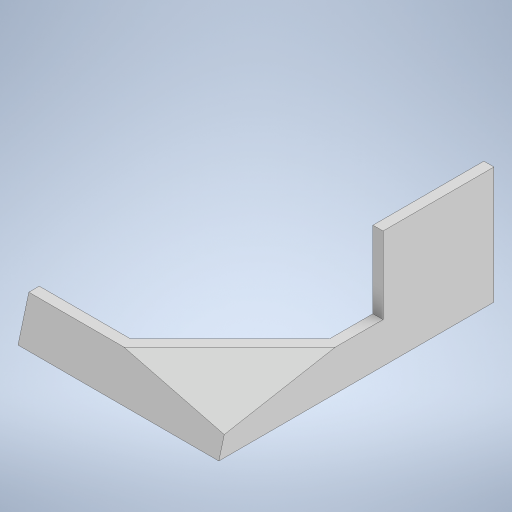
# Autodesk Inventor part: body
Saved by Autodesk Inventor 2024 (Build 280153000, 153)
## iProperties
Created: 2024-01-31
Part Number: body
Material: Všeobecné
Document SubType Name: Modeling
Designer: Simak
Density: 1 g/cm^3
Appearance: Výchozí
Author: Simak
Autodesk Inventor part; units mm, degrees
ref_plane "YZ Plane" through (0, 0, 0) normal (1, 0, 0) x (0, 1, 0)
ref_plane "XZ Plane" through (0, 0, 0) normal (0, 1, 0) x (-1, 0, 0)
ref_plane "XY Plane" through (0, 0, 0) normal (0, 0, 1) x (1, 0, 0)
sketch "Náčrt2" plane through (0, 0, 0) normal (0, 1, 0) x (-1, 0, 0)
  line L0 (0, 49.75) -> (-49.75, 49.75)
  line L1 (-49.75, 49.75) -> (-49.75, -49.75)
  line L2 (-49.75, -49.75) -> (0, -49.75)
  line L3 (-49.75, 49.75) -> (0, 0) construction
  line L4 (0, 0) -> (-49.75, -49.75) construction
  line L5 (-47.25, 49.75) -> (-47.25, -19.75)
  line L6 (-47.25, -19.75) -> (-49.75, -19.75)
  line L7 (0, 49.75) -> (0, -49.75)
  dimension "d0" = 99.5
  dimension "d1" = 69.5
  dimension "d2" = 2.5
  constraints: 16 end point, 5 perpendicular, 2 point on line, 2 vertical, 2 vertical alignment, 1 horizontal
  measures "d0" distance of L0.end L1.end
  measures "d1" distance of L5.start L5.end
  measures "d2" distance of L5.end L6.end
extrude "Vysunutí1" add sketch "Náčrt2" along normal blind 10 contours L5 L6 L1 L0
sketch "Náčrt3" plane through (49.75, 0, 49.75) normal (1, 0, 0) x (0, 0, -1)
  line L0 (69.5, 0) -> (0, 0) projected
  line L1 (69.5, 10) -> (0, 10) projected
  line L2 (0, 0) -> (0, 10) projected
  line L3 (0, 0) -> (0, -5)
  line L4 (0, -5) -> (69.5, -5) construction
  line L5 (69.5, -5) -> (69.5, 0) construction
  line L6 (0, -5) -> (4.0192, 10)
  point P0 (49.75, 0)
  point P1 (1.3397, 0)
  dimension "d8" = 5
  dimension "d9" = 75
  constraints: 8 end point, 2 perpendicular, 1 point on line, 1 vertical
  measures "d8" distance of L4.end L0.start
  measures "d9" angle of L4 L6
extrude "Vysunutí2" cut sketch "Náčrt3" against normal blind 10 contours L0 L2 L1 L6
sketch "Náčrt4" plane through (49.75, 0, -19.75) normal (1, 0, 0) x (0, 0, -1)
  line L0 (0, 10) -> (-65.4808, 10) projected
  line L1 (-62.8926, 10) -> (-65.5721, 0)
  line L2 (0, 0) -> (-68.1603, 0) projected
  line L3 (-65.4808, 10) -> (-68.1603, 0) projected
  point P0 (-19.75, 0)
  dimension "d10" = 2.5
  constraints: 2 end point, 2 point on line, 1 parallel
  measures "d10" distance between parallel lines of L3 L1
extrude "Vysunutí3" add sketch "Náčrt4" against normal up to surface (49.75 mm away)
sketch "Náčrt5" plane through (49.75, 0, -19.75) normal (1, 0, 0) x (0, 0, -1)
  line L0 (-65.4808, 10) -> (0, 10) projected
  line L1 (-27.4808, 10) -> (0, 10)
  line L2 (0, 10) -> (0, 29)
  line L3 (0, 29) -> (-27.4808, 29)
  line L4 (-27.4808, 29) -> (-27.4808, 10)
  point P0 (-19.75, 0)
  dimension "d13" = 38
  dimension "d14" = 19
  constraints: 8 end point, 2 parallel, 1 horizontal, 1 perpendicular, 1 point on line
  measures "d13" distance from line of L4 L0.start
  measures "d14" distance of L3.end L1.start
extrude "Vysunutí4" add sketch "Náčrt5" against normal up to surface (2.5 mm away)
sketch "Náčrt6" plane through (47.25, 0, -19.75) normal (-1, 0, 0) x (0, 0, 1)
  line L0 (65.5721, 0) -> (62.8926, 10) projected
  line L1 (57.5721, 1) -> (65.5721, 1)
  line L2 (65.5721, 1) -> (65.5721, 0)
  line L3 (65.5721, 0) -> (57.5721, 0)
  line L4 (57.5721, 0) -> (57.5721, 1)
  point P0 (19.75, 0)
  dimension "d17" = 1
  dimension "d18" = 8
  constraints: 8 end point, 2 parallel, 1 horizontal, 1 perpendicular
  measures "d17" distance of L3.end L1.start
  measures "d18" distance of L1.start L1.end
extrude "Vysunutí5" add sketch "Náčrt6" along normal up to surface (47.25 mm away)
sketch "Náčrt7" plane through (47.25, 0, -19.75) normal (-1, 0, 0) x (0, 0, 1)
  line L0 (62.8926, 10) -> (65.3041, 1) projected
  line L1 (64.7682, 3) -> (65.3041, 3)
  line L2 (65.3041, 3) -> (65.3041, 1)
  line L3 (65.3041, 1) -> (64.7682, 1)
  line L4 (64.7682, 1) -> (64.7682, 3)
  point P0 (19.75, 0)
  dimension "d21" = 2
  constraints: 8 end point, 2 parallel, 1 horizontal, 1 perpendicular, 1 point on line
  measures "d21" distance of L3.end L1.start
extrude "Vysunutí6" cut sketch "Náčrt7" along normal up to surface (47.25 mm away) contours L1 L2 L0
sketch "Náčrt8" plane through (0, 10, 0) normal (0, 1, 0) x (1, 0, 0)
  line L0 (49.75, -45.7308) -> (49.75, -7.7308) projected
  point P0 (0, 0)
  point P1 (23.5355, -45.7308)
  point P2 (49.75, -19.5163)
  dimension "d24" = 26.2145
  dimension "d25" = 26.2145
  constraints: 1 horizontal alignment, 1 point on line, 1 vertical alignment
  measures "d24" distance from line of L0 point (23.536, -45.731)
  measures "d25" distance of L0.start point (49.75, -19.516)
sketch "Náčrt9" plane through (49.75, 0, 48.4103) normal (1, 0, 0) x (0, 0, -1)
  line L0 (1.3397, 5) -> (0, 0) construction
  line L1 (2.6795, 10) -> (5.2677, 10) projected
  line L2 (1.3397, 5) -> (2.6795, 10) construction
  point P0 (48.4103, 0)
  constraints: 4 end point, 2 collinear
ref_plane "Pracovní rovina1" through (23.5355, 10, 45.7308) normal (-0.1757652, -0.9686141, -0.1757652) x (0.7071068, 0, -0.7071068)
sketch "Náčrt10" plane through (23.5355, 10, 45.7308) normal (-0.1757652, -0.9686141, -0.1757652) x (0.7071068, 0, -0.7071068)
  line L0 (18.5364, 17.9546) -> (-16.6421, -16.1198) projected
  line L1 (0, 0) -> (17.5891, 20.1151)
  line L2 (18.5364, 17.9546) -> (16.6417, 22.2756) projected
  line L3 (17.5891, 20.1151) -> (37.0729, 0)
  line L4 (0, 0) -> (37.0729, 0)
  point P0 (15.6944, -44.9557)
  point P1 (37.0729, 0)
  constraints: 6 end point, 1 coincident, 1 horizontal, 1 midpoint
extrude "Vysunutí7" cut sketch "Náčrt10" against normal blind 10
sketch "Náčrt11" plane through (23.5355, 10, 45.7308) normal (0.1757652, 0.9686141, 0.1757652) x (0.6849136, -0.2485695, 0.6849136)
  line L0 (0, 3.6603) -> (16.2108, 17.8353) projected
  line L1 (0, 0) -> (0, 3.6603) projected
  line L2 (20.1151, 17.5891) -> (0, 0) projected
  line L3 (0, 37.0729) -> (20.1151, 17.5891) projected
  line L4 (0, 33.5373) -> (0, 37.0729) projected
  line L5 (16.2108, 17.8353) -> (0, 33.5373) projected
  line L6 (0, 3.6603) -> (0, 33.5373)
  point P0 (-44.9557, 15.6944)
  constraints: 2 end point, 1 vertical
extrude "Vysunutí8" add sketch "Náčrt11" against normal blind 1.5
sketch "Náčrt13" plane through (23.2719, 8.5471, 45.4671) normal (-0.1757652, -0.9686141, -0.1757652) x (0.7071068, 0, -0.7071068)
  line L0 (17.5269, 16.9141) -> (33.9102, 0) projected
  line L1 (2.7368, 0) -> (17.5269, 16.9141) projected
  line L2 (2.7368, 0) -> (33.9102, 0) projected
  line L3 (33.9102, 0) -> (36.2562, -2.422)
  line L4 (43.6387, -9.7844) -> (33.5373, 0) projected
  line L5 (36.2562, -2.422) -> (0.619, -2.422)
  line L6 (0.619, -2.422) -> (2.7368, 0)
  point P0 (15.6944, -44.9557)
  point P1 (39.5718, -5.8451)
  point P2 (2.7368, 0)
  point P3 (36.0378, -2.422)
  dimension "d30" = 2.422
  constraints: 6 end point, 2 collinear, 2 point on line, 1 horizontal
  measures "d30" distance between parallel lines of L2 L5
extrude "Vysunutí9" add sketch "Náčrt13" against normal up to surface contours L3 L5 L4 L2 | L2 L4 L5 L6 surface through (48.5, 10, 15) normal (0, 1, 0)
